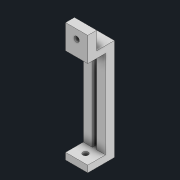
# Autodesk Inventor part: PistaSistBloq
Saved by Autodesk Inventor 2021 (Build 250183000, 183)
## iProperties
Created: 2021-05-06
Part Number: PistaSistBloq
Material: Generic
Document SubType Name: Modeling
Designer: GABRIEL LOL
Density: 1 g/cm^3
Appearance: Default
Author: GABRIEL LOL
Autodesk Inventor part; units mm, degrees
ref_plane "YZ Plane" through (0, 0, 0) normal (1, 0, 0) x (0, 1, 0)
ref_plane "XZ Plane" through (0, 0, 0) normal (0, 1, 0) x (-1, 0, 0)
ref_plane "XY Plane" through (0, 0, 0) normal (0, 0, 1) x (1, 0, 0)
sketch "Sketch1" plane through (0, 0, 0) normal (0, 0, 1) x (1, 0, 0)
  line L0 (0, 0) -> (12.5, 0)
  line L1 (12.5, 0) -> (12.5, 5)
  line L2 (12.5, 5) -> (0, 5)
  line L3 (0, 5) -> (0, 0)
  line L4 (0, 0) -> (5, 0) construction
  line L5 (12.5, 0) -> (7.5, 0) construction
  line L6 (0, 0) -> (5, 0) construction
  line L7 (5, 0) -> (5, -49.5) construction
  line L8 (5, -49.5) -> (0, -49.5) construction
  line L9 (0, -49.5) -> (0, 0) construction
  line L10 (0, 0) -> (5, 0)
  line L11 (5, 0) -> (5, -49.5)
  line L12 (5, -49.5) -> (0, -49.5)
  line L13 (0, -49.5) -> (0, 0)
  line L14 (7.5, 0) -> (12.5, 0)
  line L15 (12.5, 0) -> (12.5, -49.5)
  line L16 (12.5, -49.5) -> (7.5, -49.5)
  line L17 (7.5, -49.5) -> (7.5, 0)
  dimension "d0" = 12.5
  dimension "d1" = 5
  dimension "d2" = 5
  dimension "d3" = 5
  dimension "d4" = 49.5
  constraints: 36 end point, 8 parallel, 4 horizontal, 4 perpendicular, 3 point on line
  measures "d0" distance of L2.end L1.end
  measures "d1" distance of L1.end L0.end
  measures "d2" distance of L0.start L4.end
  measures "d3" distance of L0.end L5.end
  measures "d4" distance of L6.end L7.end
extrude "Extrusion1" add sketch "Sketch1" along normal blind 5 contours L0 L11 L12 L13 | L0 L15 L16 L17
sketch "Sketch2" plane through (0, 0, 0) normal (0, 0, -1) x (-1, 0, 0)
  line L0 (-12.5, -49.5) -> (-12.5, 0) projected
  line L1 (-7.5, -49.5) -> (-12.5, -49.5) projected
  line L2 (-7.5, 0) -> (-7.5, -49.5) projected
  line L3 (-12.5, 0) -> (-7.5, 0) projected
  line L4 (0, -49.5) -> (-5, -49.5) projected
  line L5 (0, 0) -> (0, -49.5) projected
  line L6 (-5, 0) -> (0, 0) projected
  line L7 (-5, -49.5) -> (-5, 0) projected
  line L8 (-12.5, 0) -> (0, 0)
  line L9 (0, 0) -> (0, 3.75)
  line L10 (0, 3.75) -> (-12.5, 3.75)
  line L11 (-12.5, 3.75) -> (-12.5, 0)
  line L12 (0, -49.5) -> (-5, -49.5) projected
  line L13 (0, -49.5) -> (-12.5, -49.5)
  line L14 (-12.5, -49.5) -> (-12.5, -53.25)
  line L15 (-12.5, -53.25) -> (0, -53.25)
  line L16 (0, -53.25) -> (0, -49.5)
  point P0 (-5, -49.5)
  point P1 (-7.5, -49.5)
  dimension "d7" = 3.75
  dimension "d10" = 3.75
  constraints: 16 end point, 4 parallel, 2 horizontal, 2 perpendicular
  measures "d7" distance of L9.end L8.end
  measures "d10" distance of L14.end L13.end
extrude "Extrusion2" add sketch "Sketch2" against normal blind 15 contours L1 L13 L4 L16 L15 L14 | L11 L10 L9 L6 L8 L3
sketch "Sketch4" plane through (0, -53.25, 0) normal (0, -1, 0) x (1, 0, 0)
  line L0 (7.5, 5) -> (12.5, 5) projected
  line L1 (0, 5) -> (5, 5) projected
  line L2 (12.5, 5) -> (12.5, 15) construction
  line L3 (12.5, 0) -> (0, 0) construction
  line L4 (12.5, 15) -> (0, 15) construction
  line L5 (0, 15) -> (0, 0) construction
  line L6 (0, 0) -> (12.5, 0) construction
  line L7 (12.5, 0) -> (12.5, 15) construction
  line L8 (12.5, 15) -> (0, 15) construction
  line L9 (0, 5) -> (12.5, 5) construction
  line L10 (12.5, 5) -> (12.5, 15) construction
  line L11 (12.5, 15) -> (0, 15) construction
  line L12 (0, 15) -> (0, 5) construction
  circle A0 centre (6.25, 10) radius 1.5
  dimension "d12" = 3
  constraints: 16 end point, 4 parallel, 2 horizontal, 2 perpendicular, 1 centre point
  measures "d12" diameter of A0
extrude "Extrusion3" cut sketch "Sketch4" against normal blind 10
sketch "Sketch5" plane through (0, 3.75, 0) normal (0, 1, 0) x (1, 0, 0)
  line L0 (5, -5) -> (0, -5) projected
  line L1 (12.5, -5) -> (7.5, -5) projected
  line L2 (0, 0) -> (12.5, 0) projected
  line L3 (0, 0) -> (0, -15) projected
  line L4 (12.5, -15) -> (0, -15) projected
  line L5 (12.5, 0) -> (12.5, -15) projected
  line L6 (0, 0) -> (0, -15) construction
  line L7 (7.5, -5) -> (12.5, -5) construction
  line L8 (0, 0) -> (12.5, 0) construction
  line L9 (12.5, 0) -> (12.5, -5) construction
  line L10 (12.5, -5) -> (0, -5) construction
  line L11 (0, -5) -> (0, 0) construction
  line L12 (12.5, 0) -> (12.5, -15) projected
  line L13 (12.5, -15) -> (0, -15)
  line L14 (0, -15) -> (0, -10)
  line L15 (0, -10) -> (12.5, -10)
  line L16 (12.5, -10) -> (12.5, -15)
  point P0 (0, -10)
  dimension "d15" = 12.5
  dimension "d16" = 15
  dimension "d17" = 5
  dimension "d18" = 5
  constraints: 16 end point, 4 parallel, 2 horizontal, 2 perpendicular, 1 point on line
  measures "d15" distance of L2.start L2.end
  measures "d16" distance of L2.end L4.start
  measures "d17" distance between parallel lines of L2 L1
  measures "d18" distance of L13.end L14.end
extrude "Extrusion4" add sketch "Sketch5" along normal blind 10 contours L15 L5 L4 L3
sketch "Sketch6" plane through (0, 0, 15) normal (0, 0, 1) x (1, 0, 0)
  line L0 (0, 3.75) -> (12.5, 3.75) projected
  line L1 (0, 13.75) -> (12.5, 13.75) projected
  line L2 (0, 0) -> (0, 13.75) construction
  line L3 (0, 3.75) -> (12.5, 3.75) construction
  line L4 (0, 13.75) -> (12.5, 13.75) construction
  line L5 (12.5, 13.75) -> (12.5, 3.75) construction
  line L6 (12.5, 3.75) -> (0, 3.75) construction
  line L7 (0, 3.75) -> (0, 13.75) construction
  circle A0 centre (6.25, 8.75) radius 1.5
  dimension "d21" = 3
  constraints: 8 end point, 2 parallel, 1 centre point, 1 horizontal, 1 perpendicular
  measures "d21" diameter of A0
extrude "Extrusion5" cut sketch "Sketch6" against normal blind 10
body "Solid1"
